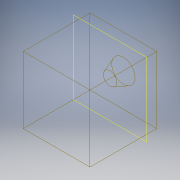
# Autodesk Inventor part: hako
Saved by Autodesk Inventor 2019.1 (Build 231200000, 200)
## iProperties
Created: 2018-12-21
Part Number: hako
Material: アルミニウム 6061
Document SubType Name: Modeling
Designer: Masaya
Density: 2.7 g/cm^3
Appearance: メタル 2400F 熱
Author: Masaya
Autodesk Inventor part; units mm, degrees
ref_plane "YZ Plane" through (0, 0, 0) normal (1, 0, 0) x (0, 1, 0)
ref_plane "XZ Plane" through (0, 0, 0) normal (0, 1, 0) x (-1, 0, 0)
ref_plane "XY Plane" through (0, 0, 0) normal (0, 0, 1) x (1, 0, 0)
sketch "スケッチ1" plane through (0, 0, 0) normal (0, 1, 0) x (-1, 0, 0)
  line L0 (2000, 2000) -> (0, 2000)
  line L1 (0, 2000) -> (0, 0)
  line L2 (0, 0) -> (2000, 0)
  line L3 (2000, 0) -> (2000, 2000)
  dimension "d0" = 2000
  dimension "d1" = 2000
  constraints: 8 end point, 2 parallel, 1 coincident, 1 horizontal, 1 perpendicular
  measures "d0" distance of L2.end L1.end
  measures "d1" distance of L1.end L0.end
extrude "押し出し1" add sketch "スケッチ1" along normal blind 2000
sketch "スケッチ2" plane through (0, 0, 0) normal (0, 0, -1) x (-1, 0, 0)
  circle A0 centre (1000, 1000) radius 350
  line L0 (2000, 2000) -> (0, 2000) construction
  line L1 (1000, 2000) -> (1000, 1000) construction
  line L2 (1000, 1000) -> (2000, 1000) construction
  line L3 (2000, 0) -> (2000, 2000) construction
  point P0 (0, 0)
  dimension "d4" = 700
  constraints: 4 end point, 2 midpoint, 1 centre point, 1 coincident, 1 perpendicular, 1 vertical
  measures "d4" diameter of A0
ref_plane "作業平面1" through (0, 0, 400) normal (0, 0, -1) x (-1, 0, 0)
sketch "スケッチ3" plane through (0, 0, 400) normal (0, 0, -1) x (-1, 0, 0)
  circle A0 centre (1000, 1000) radius 200
  point P0 (0, 0)
  dimension "d6" = 400
  constraints: 1 centre point, 1 coincident
  measures "d6" diameter of A0
loft "ロフト1" cut profiles "スケッチ2", "スケッチ3"
